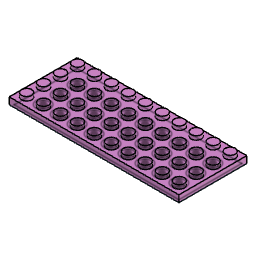
lego_4x10 (Autodesk Fusion 360 design; units mm, degrees)
Autodesk Fusion 360 part; units mm, degrees
sketch "Skizze1" plane through (0, 0, 0) normal (0, 0, 1) x (1, 0, 0)
  line L0 (40, -16) -> (-40, -16)
  line L1 (-40, -16) -> (-40, 16)
  line L2 (-40, 16) -> (40, 16)
  line L3 (40, 16) -> (40, -16)
  line L4 (40, -16) -> (-40, 16) construction
  line L5 (-40, -16) -> (40, 16) construction
  dimension "d1" = 80
  dimension "d2" = 32
  constraint horizontal L0
  constraint perpendicular L0 L1
  constraint parallel L0 L2
  constraint parallel L1 L3
  constraint coincident L4 origin
  constraint coincident L5 origin
  measures "d1" distance of L1.end L2.end
  measures "d2" distance of L0.end L1.end
extrude "Extrusion1" add sketch "Skizze1" along normal blind 3.2
sketch "Skizze2" plane through (0, 0, 3.2) normal (0, 0, 1) x (-1, 0, 0)
  line L0 (-40, -16) -> (40, -16)
  line L1 (40, -16) -> (40, 16)
  line L2 (40, 16) -> (-40, 16)
  line L3 (-40, 16) -> (-40, -16)
  circle A0 centre (-36.1, -12.1) radius 2.4
  circle A1 centre (-28.1, -12.1) radius 2.4
  circle A2 centre (-20.1, -12.1) radius 2.4
  circle A3 centre (-12.1, -12.1) radius 2.4
  circle A4 centre (-4.1, -12.1) radius 2.4
  circle A5 centre (3.9, -12.1) radius 2.4
  circle A6 centre (11.9, -12.1) radius 2.4
  circle A7 centre (19.9, -12.1) radius 2.4
  circle A8 centre (27.9, -12.1) radius 2.4
  circle A9 centre (35.9, -12.1) radius 2.4
  circle A10 centre (-36.1, -4.1) radius 2.4
  circle A11 centre (-28.1, -4.1) radius 2.4
  circle A12 centre (-20.1, -4.1) radius 2.4
  circle A13 centre (-12.1, -4.1) radius 2.4
  circle A14 centre (-4.1, -4.1) radius 2.4
  circle A15 centre (3.9, -4.1) radius 2.4
  circle A16 centre (11.9, -4.1) radius 2.4
  circle A17 centre (19.9, -4.1) radius 2.4
  circle A18 centre (27.9, -4.1) radius 2.4
  circle A19 centre (35.9, -4.1) radius 2.4
  circle A20 centre (-36.1, 3.9) radius 2.4
  circle A21 centre (-28.1, 3.9) radius 2.4
  circle A22 centre (-20.1, 3.9) radius 2.4
  circle A23 centre (-12.1, 3.9) radius 2.4
  circle A24 centre (-4.1, 3.9) radius 2.4
  circle A25 centre (3.9, 3.9) radius 2.4
  circle A26 centre (11.9, 3.9) radius 2.4
  circle A27 centre (19.9, 3.9) radius 2.4
  circle A28 centre (27.9, 3.9) radius 2.4
  circle A29 centre (35.9, 3.9) radius 2.4
  circle A30 centre (-36.1, 11.9) radius 2.4
  circle A31 centre (-28.1, 11.9) radius 2.4
  circle A32 centre (-20.1, 11.9) radius 2.4
  circle A33 centre (-12.1, 11.9) radius 2.4
  circle A34 centre (-4.1, 11.9) radius 2.4
  circle A35 centre (3.9, 11.9) radius 2.4
  circle A36 centre (11.9, 11.9) radius 2.4
  circle A37 centre (19.9, 11.9) radius 2.4
  circle A38 centre (27.9, 11.9) radius 2.4
  circle A39 centre (35.9, 11.9) radius 2.4
  dimension "d5" = 4.8
  dimension "d6" = 3.9
  dimension "d7" = 3.9
  dimension "d10" = 8
  dimension "d11" = 8
  measures "d5" diameter of A0
  measures "d6" distance of L3 A0.centre
  measures "d7" distance of L0 A0.centre
extrude "Extrusion2" add sketch "Skizze2" along normal blind 1.8 contours A0 | A1 | A2 | A3 | A4 | A5 | A6 | A7 | A8 | A9 | A10 | A11 | A12 | A13 | A14 | A15 | A16 | A17 | A18 | A19 | A20 | A21 | A22 | A23 | A24 | A25 | A26 | A27 | A28 | A29 | A30 | A31 | A32 | A33 | A34 | A35 | A36 | A37 | A38 | A39
sketch "Skizze3" plane through (0, 0, 0) normal (0, 0, -1) x (1, 0, 0)
  line L0 (-40, -16) -> (40, -16)
  line L1 (40, -16) -> (40, 16)
  line L2 (40, 16) -> (-40, 16)
  line L3 (-40, 16) -> (-40, -16)
  circle A0 centre (-32.1, -8.1) radius 3.255
  circle A1 centre (-32.1, -8.1) radius 2.4
  circle A2 centre (-24.1, -8.1) radius 2.4
  circle A3 centre (-24.1, -8.1) radius 3.255
  circle A4 centre (-16.1, -8.1) radius 2.4
  circle A5 centre (-16.1, -8.1) radius 3.255
  circle A6 centre (-8.1, -8.1) radius 2.4
  circle A7 centre (-8.1, -8.1) radius 3.255
  circle A8 centre (-0.1, -8.1) radius 2.4
  circle A9 centre (-0.1, -8.1) radius 3.255
  circle A10 centre (7.9, -8.1) radius 2.4
  circle A11 centre (7.9, -8.1) radius 3.255
  circle A12 centre (15.9, -8.1) radius 2.4
  circle A13 centre (15.9, -8.1) radius 3.255
  circle A14 centre (23.9, -8.1) radius 2.4
  circle A15 centre (23.9, -8.1) radius 3.255
  circle A16 centre (31.9, -8.1) radius 2.4
  circle A17 centre (31.9, -8.1) radius 3.255
  circle A18 centre (-32.1, -0.1) radius 2.4
  circle A19 centre (-32.1, -0.1) radius 3.255
  circle A20 centre (-24.1, -0.1) radius 2.4
  circle A21 centre (-24.1, -0.1) radius 3.255
  circle A22 centre (-16.1, -0.1) radius 2.4
  circle A23 centre (-16.1, -0.1) radius 3.255
  circle A24 centre (-8.1, -0.1) radius 2.4
  circle A25 centre (-8.1, -0.1) radius 3.255
  circle A26 centre (-0.1, -0.1) radius 2.4
  circle A27 centre (-0.1, -0.1) radius 3.255
  circle A28 centre (7.9, -0.1) radius 2.4
  circle A29 centre (7.9, -0.1) radius 3.255
  circle A30 centre (15.9, -0.1) radius 2.4
  circle A31 centre (15.9, -0.1) radius 3.255
  circle A32 centre (23.9, -0.1) radius 2.4
  circle A33 centre (23.9, -0.1) radius 3.255
  circle A34 centre (31.9, -0.1) radius 2.4
  circle A35 centre (31.9, -0.1) radius 3.255
  circle A36 centre (-32.1, 7.9) radius 2.4
  circle A37 centre (-32.1, 7.9) radius 3.255
  circle A38 centre (-24.1, 7.9) radius 2.4
  circle A39 centre (-24.1, 7.9) radius 3.255
  circle A40 centre (-16.1, 7.9) radius 2.4
  circle A41 centre (-16.1, 7.9) radius 3.255
  circle A42 centre (-8.1, 7.9) radius 2.4
  circle A43 centre (-8.1, 7.9) radius 3.255
  circle A44 centre (-0.1, 7.9) radius 2.4
  circle A45 centre (-0.1, 7.9) radius 3.255
  circle A46 centre (7.9, 7.9) radius 2.4
  circle A47 centre (7.9, 7.9) radius 3.255
  circle A48 centre (15.9, 7.9) radius 2.4
  circle A49 centre (15.9, 7.9) radius 3.255
  circle A50 centre (23.9, 7.9) radius 2.4
  circle A51 centre (23.9, 7.9) radius 3.255
  circle A52 centre (31.9, 7.9) radius 2.4
  circle A53 centre (31.9, 7.9) radius 3.255
  line L4 (-38.8, -14.8) -> (38.8, -14.8)
  line L5 (38.8, -14.8) -> (38.8, 14.8)
  line L6 (38.8, 14.8) -> (-38.8, 14.8)
  line L7 (-38.8, 14.8) -> (-38.8, -14.8)
  dimension "d14" = 6.51
  dimension "d15" = -0.855
  dimension "d19" = 7.9
  dimension "d20" = 7.9
  dimension "d23" = 8
  dimension "d24" = 8
  dimension "d25" = -1.2
  measures "d14" diameter of A0
  measures "d19" distance of L0 A0.centre
  measures "d20" distance of L3 A0.centre
extrude "Extrusion3" cut sketch "Skizze3" against normal blind 2.2 contours L4 L5 L6 L7
extrude "Extrusion4" cut sketch "Skizze3" against normal blind 2.2 contours A1 | A2 | A4 | A6 | A8 | A10 | A12 | A14 | A16 | A18 | A20 | A22 | A24 | A26 | A28 | A30 | A32 | A34 | A36 | A38 | A40 | A42 | A44 | A46 | A48 | A50 | A52
